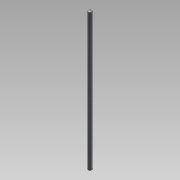
# Autodesk Inventor part: Z Akse gevindstang
Saved by Autodesk Inventor 2016 (Build 200138000, 138)
## iProperties
Created: 2015-06-04
Part Number: Z Akse gevindstang
Material: Aluminum 6061
Document SubType Name: Modeling
Designer: Mathias L. Kjeldgaard
Density: 2.71 g/cm^3
Appearance: Aluminum - Flat
Mass: 39.9834 g
Surface Area: 75.2183 cm^2
Volume: 14.754 cm^3
Author: Mathias L. Kjeldgaard
Autodesk Inventor part; units mm, degrees
ref_plane "YZ Plane" through (0, 0, 0) normal (1, 0, 0) x (0, 1, 0)
ref_plane "XZ Plane" through (0, 0, 0) normal (0, 1, 0) x (-1, 0, 0)
ref_plane "XY Plane" through (0, 0, 0) normal (0, 0, 1) x (1, 0, 0)
sketch "Sketch1" plane through (0, 0, 0) normal (0, 0, 1) x (1, 0, 0)
  circle A0 centre (0, 0) radius 4
  dimension "d0" = 8
  constraints: 1 centre point, 1 coincident
  measures "d0" diameter of A0
extrude "Extrusion1" add sketch "Sketch1" along normal mid plane 300
fillet "Fillet1" radius 2 2 edges at (-4, 0, 150) (-4, 0, -150)
thread "Thread1" size "M8x1.25" class "6g" standard "ANSI Metric M Profile" full length
sketch "Sketch2" plane through (0, 0, -150) normal (0, 0, -1) x (-1, 0, 0)
  circle A0 centre (0, 0) radius 2 construction
  circle A1 centre (0, 0) radius 4.5
  circle A2 centre (0, 0) radius 4 construction
  circle A3 centre (0, 0) radius 2.5
  dimension "d6" = 0.5
  dimension "d7" = 5
  constraints: 2 centre point, 2 coincident
  measures "d6" radial gap between concentric circles of A1 A2
  measures "d7" diameter of A3
extrude "Extrusion2" cut sketch "Sketch2" against normal blind 10
body "Solid1"
